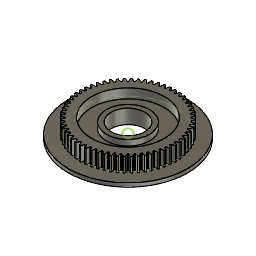
roller (Autodesk Fusion 360 design; units mm, degrees)
part number: 2025-11-25-15-03-10-225
description: Spur Gear; Module: 1.617; Num Teeth: 60; Pressure Angle: 20.0; Backlash: 0.00 mm
part number: 2025-11-25-15-09-40-850
Autodesk Fusion 360 part; units mm, degrees
(part 1 of 11)
sketch "Sketch1" plane through (0, 0, 0) normal (0, 0, 1) x (1, 0, 0) in component "Spur Gear (60 teeth)"
  circle A0 centre (0, 0) radius 46.5188
  circle A1 centre (0, 0) radius 17.65
  dimension "d15" = 35.3
  measures "d15" diameter of A1
extrude "Extrude1" add sketch "Sketch1" along normal blind 15 in component "Spur Gear (60 teeth)"
sketch "Sketch2" plane through (0, 0, 0) normal (0, 0, 1) x (1, 0, 0) in component "Spur Gear (60 teeth)"
  spline S0 degree 5 poles (45.546, -1.8723) (45.5592, -1.8723) (45.5856, -1.8721) (45.6253, -1.8716) (45.6781, -1.8704) (45.7442, -1.8678) (45.8102, -1.8642) (45.8763, -1.8596) (45.9424, -1.8541) (46.0085, -1.8477) (46.0745, -1.8406) (46.1406, -1.8328) (46.2066, -1.8243) (46.2727, -1.8154) (46.3387, -1.806) (46.4047, -1.796) (46.4707, -1.7856) (46.5367, -1.7747) (46.6026, -1.7633) (46.6686, -1.7514) (46.7345, -1.739) (46.8004, -1.7263) (46.8663, -1.7131) (46.9322, -1.6994) (46.998, -1.6854) (47.0638, -1.671) (47.1296, -1.6562) (47.1954, -1.6411) (47.2611, -1.6255) (47.3268, -1.6096) (47.3925, -1.5933) (47.4582, -1.5767) (47.5239, -1.5597) (47.5895, -1.5424) (47.6551, -1.5247) (47.7206, -1.5067) (47.7862, -1.4884) (47.8517, -1.4697) (47.9171, -1.4507) (47.9826, -1.4314) (48.048, -1.4118) (48.1134, -1.3919) (48.1787, -1.3717) (48.2441, -1.3511) (48.3093, -1.3303) (48.3746, -1.3092) (48.4398, -1.2877) (48.505, -1.266) (48.5702, -1.244) (48.6353, -1.2217) (48.7004, -1.1991) (48.7654, -1.1763) (48.8305, -1.1532) (48.8955, -1.1297) (48.9604, -1.1061) (49.0253, -1.0821) (49.0902, -1.0579) (49.155, -1.0334) (49.2198, -1.0086) (49.2846, -0.9836) (49.3493, -0.9583) (49.414, -0.9328) (49.4787, -0.907) (49.5433, -0.881) (49.6079, -0.8546) (49.6724, -0.8281) (49.7369, -0.8013) (49.8013, -0.7742) (49.8657, -0.7469) (49.9301, -0.7194) (49.9944, -0.6916) (50.0459, -0.6691) (50.0844, -0.6522) (50.1101, -0.6409) (50.123, -0.6352) knots 0 0 0 0 0 0 0.01428571 0.02857143 0.04285714 0.05714286 0.07142857 0.08571429 0.1 0.11428571 0.12857143 0.14285714 0.15714286 0.17142857 0.18571429 0.2 0.21428571 0.22857143 0.24285714 0.25714286 0.27142857 0.28571429 0.3 0.31428571 0.32857143 0.34285714 0.35714286 0.37142857 0.38571429 0.4 0.41428571 0.42857143 0.44285714 0.45714286 0.47142857 0.48571429 0.5 0.51428571 0.52857143 0.54285714 0.55714286 0.57142857 0.58571429 0.6 0.61428571 0.62857143 0.64285714 0.65714286 0.67142857 0.68571429 0.7 0.71428571 0.72857143 0.74285714 0.75714286 0.77142857 0.78571429 0.8 0.81428571 0.82857143 0.84285714 0.85714286 0.87142857 0.88571429 0.9 0.91428571 0.92857143 0.94285714 0.95714286 0.97142857 0.98571429 1 1 1 1 1 1
  spline S1 degree 5 poles (45.546, 1.8723) (45.5592, 1.8723) (45.5856, 1.8721) (45.6253, 1.8716) (45.6781, 1.8704) (45.7442, 1.8678) (45.8102, 1.8642) (45.8763, 1.8596) (45.9424, 1.8541) (46.0085, 1.8477) (46.0745, 1.8406) (46.1406, 1.8328) (46.2066, 1.8243) (46.2727, 1.8154) (46.3387, 1.806) (46.4047, 1.796) (46.4707, 1.7856) (46.5367, 1.7747) (46.6026, 1.7633) (46.6686, 1.7514) (46.7345, 1.739) (46.8004, 1.7263) (46.8663, 1.7131) (46.9322, 1.6994) (46.998, 1.6854) (47.0638, 1.671) (47.1296, 1.6562) (47.1954, 1.6411) (47.2611, 1.6255) (47.3268, 1.6096) (47.3925, 1.5933) (47.4582, 1.5767) (47.5239, 1.5597) (47.5895, 1.5424) (47.6551, 1.5247) (47.7206, 1.5067) (47.7862, 1.4884) (47.8517, 1.4697) (47.9171, 1.4507) (47.9826, 1.4314) (48.048, 1.4118) (48.1134, 1.3919) (48.1787, 1.3717) (48.2441, 1.3511) (48.3093, 1.3303) (48.3746, 1.3092) (48.4398, 1.2877) (48.505, 1.266) (48.5702, 1.244) (48.6353, 1.2217) (48.7004, 1.1991) (48.7654, 1.1763) (48.8305, 1.1532) (48.8955, 1.1297) (48.9604, 1.1061) (49.0253, 1.0821) (49.0902, 1.0579) (49.155, 1.0334) (49.2198, 1.0086) (49.2846, 0.9836) (49.3493, 0.9583) (49.414, 0.9328) (49.4787, 0.907) (49.5433, 0.881) (49.6079, 0.8546) (49.6724, 0.8281) (49.7369, 0.8013) (49.8013, 0.7742) (49.8657, 0.7469) (49.9301, 0.7194) (49.9944, 0.6916) (50.0459, 0.6691) (50.0844, 0.6522) (50.1101, 0.6409) (50.123, 0.6352) knots 0 0 0 0 0 0 0.01428571 0.02857143 0.04285714 0.05714286 0.07142857 0.08571429 0.1 0.11428571 0.12857143 0.14285714 0.15714286 0.17142857 0.18571429 0.2 0.21428571 0.22857143 0.24285714 0.25714286 0.27142857 0.28571429 0.3 0.31428571 0.32857143 0.34285714 0.35714286 0.37142857 0.38571429 0.4 0.41428571 0.42857143 0.44285714 0.45714286 0.47142857 0.48571429 0.5 0.51428571 0.52857143 0.54285714 0.55714286 0.57142857 0.58571429 0.6 0.61428571 0.62857143 0.64285714 0.65714286 0.67142857 0.68571429 0.7 0.71428571 0.72857143 0.74285714 0.75714286 0.77142857 0.78571429 0.8 0.81428571 0.82857143 0.84285714 0.85714286 0.87142857 0.88571429 0.9 0.91428571 0.92857143 0.94285714 0.95714286 0.97142857 0.98571429 1 1 1 1 1 1
  arc A0 (50.123, -0.6352) -> (50.123, 0.6352) centre (0, 0) ccw
  line L0 (45.546, 1.8723) -> (45.546, -1.8723)
  point P0 (45.8713, -1.8597)
  point P1 (46.1974, -1.8254)
  point P2 (46.524, -1.7767)
  point P3 (46.8509, -1.7161)
  point P4 (47.1781, -1.645)
  point P5 (47.5055, -1.5644)
  point P6 (47.833, -1.475)
  point P7 (48.1605, -1.3772)
  point P8 (48.488, -1.2716)
  point P9 (48.8154, -1.1585)
  point P10 (49.1426, -1.038)
  point P11 (49.4697, -0.9105)
  point P12 (49.7965, -0.7762)
  point P13 (45.8713, 1.8597)
  point P14 (46.1974, 1.8254)
  point P15 (46.524, 1.7767)
  point P16 (46.8509, 1.7161)
  point P17 (47.1781, 1.645)
  point P18 (47.5055, 1.5644)
  point P19 (47.833, 1.475)
  point P20 (48.1605, 1.3772)
  point P21 (48.488, 1.2716)
  point P22 (48.8154, 1.1585)
  point P23 (49.1426, 1.038)
  point P24 (49.4697, 0.9105)
  point P25 (49.7965, 0.7762)
extrude "Extrude2" add sketch "Sketch2" along normal blind 15 in component "Spur Gear (60 teeth)"
fillet "Fillet1" radius 0.4 2 edges at (46.4846, 1.7832, 7.5) (46.4846, -1.7832, 7.5) in component "Spur Gear (60 teeth)"
pattern_circular "C-Pattern1" count 60 over 360 about axis through (0, 0, 0) along (0, 0, 1) of "Extrude2", "Fillet1" in component "Spur Gear (60 teeth)"
sketch "Sketch3" plane through (0, 0, 0) normal (0, 0, 1) x (1, 0, 0) in component "Spur Gear (60 teeth)"
  circle A0 centre (0, 0) radius 48.51 construction
sketch "Sketch1 (2)" plane through (0, 0, 0) normal (0, 0, -1) x (1, 0, 0)
  circle A0 centre (0, 0) radius 17.65
  spline S0 degree 3 poles (46.1303, 8.0392) (46.0824, 8.0188) (46.039, 7.9892) (45.9659, 7.915) (45.9369, 7.8711) (45.9032, 7.7887) (45.894, 7.7528) (45.8858, 7.6794) (45.8868, 7.6424) (45.8928, 7.606) knots 0 0 0 0 0.015626 0.015626 0.031252 0.031252 0.042323 0.042323 0.053393 0.053393 0.053393 0.053393
  spline S1 degree 5 poles (46.1303, 8.0392) (46.1316, 8.0398) (46.1452, 8.0456) (46.1711, 8.0567) (46.2094, 8.0733) (46.2599, 8.0954) (46.3214, 8.1228) (46.3828, 8.1506) (46.4441, 8.1788) (46.5052, 8.2073) (46.5663, 8.2361) (46.6273, 8.2654) (46.6882, 8.295) (46.7489, 8.3249) (46.8096, 8.3552) (46.8702, 8.3857) (46.9307, 8.4167) (46.9911, 8.4479) (47.0514, 8.4795) (47.1116, 8.5113) (47.1717, 8.5435) (47.2317, 8.576) (47.2916, 8.6088) (47.3514, 8.6419) (47.4111, 8.6752) (47.4707, 8.7089) (47.5303, 8.7429) (47.5897, 8.7771) (47.649, 8.8116) (47.7083, 8.8464) (47.7674, 8.8815) (47.8265, 8.9168) (47.8855, 8.9524) (47.9444, 8.9883) (48.0032, 9.0245) (48.0619, 9.0609) (48.1205, 9.0975) (48.179, 9.1345) (48.2374, 9.1717) (48.2957, 9.2091) (48.354, 9.2468) (48.4121, 9.2847) (48.4702, 9.3229) (48.5281, 9.3613) (48.586, 9.4) (48.6438, 9.4389) (48.7015, 9.4781) (48.7591, 9.5175) (48.8166, 9.5571) (48.874, 9.597) (48.9314, 9.6371) (48.9886, 9.6774) (49.0457, 9.718) (49.0914, 9.7506) (49.1256, 9.7752) (49.1483, 9.7916) (49.1597, 9.7998) knots 0.269981 0.269981 0.269981 0.269981 0.269981 0.269981 0.271429 0.285714 0.3 0.314286 0.328571 0.342857 0.357143 0.371429 0.385714 0.4 0.414286 0.428571 0.442857 0.457143 0.471429 0.485714 0.5 0.514286 0.528571 0.542857 0.557143 0.571429 0.585714 0.6 0.614286 0.628571 0.642857 0.657143 0.671429 0.685714 0.7 0.714286 0.728571 0.742857 0.757143 0.771429 0.785714 0.8 0.814286 0.828571 0.842857 0.857143 0.871429 0.885714 0.9 0.914286 0.928571 0.942857 0.957143 0.971429 0.985714 1 1 1 1 1 1
  arc A1 (49.1597, 9.7998) -> (48.8956, 11.0425) centre (0, 0) ccw
  spline S2 degree 5 poles (45.412, 11.4187) (45.4134, 11.4187) (45.4282, 11.4189) (45.4564, 11.4193) (45.4981, 11.4197) (45.5532, 11.42) (45.6206, 11.42) (45.6879, 11.4196) (45.7554, 11.4188) (45.8229, 11.4177) (45.8904, 11.4161) (45.958, 11.4142) (46.0256, 11.412) (46.0933, 11.4093) (46.1611, 11.4064) (46.2289, 11.4031) (46.2967, 11.3994) (46.3646, 11.3954) (46.4325, 11.3911) (46.5004, 11.3865) (46.5684, 11.3816) (46.6364, 11.3763) (46.7045, 11.3707) (46.7726, 11.3648) (46.8407, 11.3586) (46.9089, 11.3521) (46.9771, 11.3453) (47.0453, 11.3382) (47.1136, 11.3308) (47.1818, 11.3231) (47.2502, 11.3151) (47.3185, 11.3069) (47.3869, 11.2983) (47.4552, 11.2895) (47.5237, 11.2804) (47.5921, 11.271) (47.6605, 11.2613) (47.729, 11.2514) (47.7975, 11.2412) (47.866, 11.2307) (47.9346, 11.22) (48.0031, 11.209) (48.0717, 11.1977) (48.1403, 11.1862) (48.2089, 11.1744) (48.2775, 11.1623) (48.3461, 11.15) (48.4148, 11.1375) (48.4834, 11.1246) (48.5521, 11.1116) (48.6208, 11.0983) (48.6895, 11.0847) (48.7582, 11.0709) (48.8131, 11.0596) (48.8544, 11.0511) (48.8819, 11.0453) (48.8956, 11.0425) knots 0.269981 0.269981 0.269981 0.269981 0.269981 0.269981 0.271429 0.285714 0.3 0.314286 0.328571 0.342857 0.357143 0.371429 0.385714 0.4 0.414286 0.428571 0.442857 0.457143 0.471429 0.485714 0.5 0.514286 0.528571 0.542857 0.557143 0.571429 0.585714 0.6 0.614286 0.628571 0.642857 0.657143 0.671429 0.685714 0.7 0.714286 0.728571 0.742857 0.757143 0.771429 0.785714 0.8 0.814286 0.828571 0.842857 0.857143 0.871429 0.885714 0.9 0.914286 0.928571 0.942857 0.957143 0.971429 0.985714 1 1 1 1 1 1
  spline S3 degree 3 poles (45.0188, 11.7179) (45.0319, 11.6675) (45.0547, 11.6201) (45.1173, 11.5368) (45.1564, 11.5017) (45.2328, 11.4561) (45.267, 11.4417) (45.3383, 11.4227) (45.3751, 11.4181) (45.412, 11.4187) knots 0 0 0 0 0.015626 0.015626 0.031252 0.031252 0.042323 0.042323 0.053393 0.053393 0.053393 0.053393
  arc A2 (45.0188, 11.7179) -> (44.8463, 12.3614) centre (0, 0) ccw
  spline S4 degree 3 poles (45.0373, 12.8171) (44.9918, 12.7918) (44.9517, 12.7578) (44.8867, 12.6763) (44.8625, 12.6297) (44.8376, 12.5442) (44.8322, 12.5076) (44.8317, 12.4337) (44.8365, 12.397) (44.8463, 12.3614) knots 0 0 0 0 0.015626 0.015626 0.031252 0.031252 0.042323 0.042323 0.053393 0.053393 0.053393 0.053393
  spline S5 degree 5 poles (45.0373, 12.8171) (45.0385, 12.8178) (45.0514, 12.825) (45.076, 12.8388) (45.1124, 12.8593) (45.1603, 12.8866) (45.2186, 12.9202) (45.2767, 12.9543) (45.3347, 12.9887) (45.3926, 13.0234) (45.4503, 13.0585) (45.5079, 13.094) (45.5654, 13.1298) (45.6227, 13.1659) (45.6798, 13.2023) (45.7369, 13.2391) (45.7938, 13.2762) (45.8506, 13.3135) (45.9073, 13.3512) (45.9638, 13.3892) (46.0202, 13.4275) (46.0765, 13.4661) (46.1326, 13.5049) (46.1887, 13.5441) (46.2446, 13.5835) (46.3003, 13.6232) (46.356, 13.6632) (46.4115, 13.7035) (46.4669, 13.744) (46.5222, 13.7848) (46.5774, 13.8259) (46.6325, 13.8672) (46.6874, 13.9088) (46.7422, 13.9506) (46.7969, 13.9927) (46.8515, 14.0351) (46.9059, 14.0777) (46.9602, 14.1205) (47.0145, 14.1636) (47.0686, 14.2069) (47.1225, 14.2505) (47.1764, 14.2943) (47.2301, 14.3383) (47.2838, 14.3826) (47.3373, 14.4271) (47.3907, 14.4719) (47.444, 14.5169) (47.4971, 14.5621) (47.5502, 14.6075) (47.6031, 14.6531) (47.656, 14.699) (47.7087, 14.7451) (47.7613, 14.7914) (47.8032, 14.8286) (47.8347, 14.8567) (47.8556, 14.8754) (47.8661, 14.8847) knots 0.269981 0.269981 0.269981 0.269981 0.269981 0.269981 0.271429 0.285714 0.3 0.314286 0.328571 0.342857 0.357143 0.371429 0.385714 0.4 0.414286 0.428571 0.442857 0.457143 0.471429 0.485714 0.5 0.514286 0.528571 0.542857 0.557143 0.571429 0.585714 0.6 0.614286 0.628571 0.642857 0.657143 0.671429 0.685714 0.7 0.714286 0.728571 0.742857 0.757143 0.771429 0.785714 0.8 0.814286 0.828571 0.842857 0.857143 0.871429 0.885714 0.9 0.914286 0.928571 0.942857 0.957143 0.971429 0.985714 1 1 1 1 1 1
  arc A3 (47.8661, 14.8847) -> (47.4735, 16.093) centre (0, 0) ccw
  spline S6 degree 5 poles (43.9697, 16.103) (43.971, 16.1031) (43.9857, 16.1049) (44.0137, 16.1082) (44.0551, 16.113) (44.11, 16.1191) (44.1769, 16.1261) (44.244, 16.1328) (44.3111, 16.139) (44.3784, 16.1449) (44.4457, 16.1504) (44.5131, 16.1556) (44.5806, 16.1604) (44.6482, 16.1649) (44.7159, 16.169) (44.7837, 16.1728) (44.8515, 16.1763) (44.9194, 16.1794) (44.9874, 16.1823) (45.0555, 16.1847) (45.1236, 16.1869) (45.1918, 16.1888) (45.2601, 16.1904) (45.3284, 16.1916) (45.3968, 16.1926) (45.4653, 16.1932) (45.5338, 16.1936) (45.6024, 16.1937) (45.6711, 16.1934) (45.7398, 16.1929) (45.8086, 16.1921) (45.8774, 16.1911) (45.9463, 16.1897) (46.0152, 16.1881) (46.0842, 16.1862) (46.1532, 16.184) (46.2223, 16.1815) (46.2915, 16.1788) (46.3606, 16.1758) (46.4299, 16.1726) (46.4992, 16.169) (46.5685, 16.1653) (46.6379, 16.1612) (46.7073, 16.1569) (46.7767, 16.1524) (46.8462, 16.1476) (46.9158, 16.1425) (46.9854, 16.1372) (47.055, 16.1316) (47.1246, 16.1258) (47.1943, 16.1197) (47.2641, 16.1134) (47.3338, 16.1069) (47.3897, 16.1014) (47.4316, 16.0972) (47.4595, 16.0944) (47.4735, 16.093) knots 0.269981 0.269981 0.269981 0.269981 0.269981 0.269981 0.271429 0.285714 0.3 0.314286 0.328571 0.342857 0.357143 0.371429 0.385714 0.4 0.414286 0.428571 0.442857 0.457143 0.471429 0.485714 0.5 0.514286 0.528571 0.542857 0.557143 0.571429 0.585714 0.6 0.614286 0.628571 0.642857 0.657143 0.671429 0.685714 0.7 0.714286 0.728571 0.742857 0.757143 0.771429 0.785714 0.8 0.814286 0.828571 0.842857 0.857143 0.871429 0.885714 0.9 0.914286 0.928571 0.942857 0.957143 0.971429 0.985714 1 1 1 1 1 1
  spline S7 degree 3 poles (43.5473, 16.3594) (43.5656, 16.3107) (43.5933, 16.266) (43.6642, 16.1896) (43.7068, 16.1588) (43.7876, 16.1215) (43.823, 16.1107) (43.896, 16.0992) (43.933, 16.0986) (43.9697, 16.103) knots 0 0 0 0 0.015626 0.015626 0.031252 0.031252 0.042323 0.042323 0.053393 0.053393 0.053393 0.053393
  arc A4 (43.5473, 16.3594) -> (43.3086, 16.9814) centre (0, 0) ccw
  spline S8 degree 3 poles (43.4508, 17.4546) (43.4082, 17.4246) (43.3719, 17.3866) (43.3158, 17.2988) (43.2966, 17.2499) (43.2808, 17.1623) (43.2793, 17.1253) (43.2864, 17.0518) (43.2951, 17.0158) (43.3086, 16.9814) knots 0 0 0 0 0.015626 0.015626 0.031252 0.031252 0.042323 0.042323 0.053393 0.053393 0.053393 0.053393
  spline S9 degree 5 poles (43.4508, 17.4546) (43.4519, 17.4554) (43.464, 17.4639) (43.4871, 17.4802) (43.5211, 17.5043) (43.5659, 17.5365) (43.6203, 17.5761) (43.6746, 17.616) (43.7287, 17.6563) (43.7826, 17.6969) (43.8363, 17.7378) (43.8899, 17.7791) (43.9433, 17.8207) (43.9965, 17.8626) (44.0496, 17.9048) (44.1025, 17.9474) (44.1552, 17.9902) (44.2078, 18.0333) (44.2602, 18.0767) (44.3125, 18.1204) (44.3645, 18.1644) (44.4165, 18.2086) (44.4683, 18.2531) (44.5199, 18.2979) (44.5714, 18.343) (44.6227, 18.3883) (44.6739, 18.4339) (44.7249, 18.4797) (44.7758, 18.5258) (44.8265, 18.5722) (44.8771, 18.6188) (44.9275, 18.6657) (44.9778, 18.7128) (45.0279, 18.7601) (45.0779, 18.8077) (45.1277, 18.8555) (45.1774, 18.9036) (45.227, 18.9518) (45.2764, 19.0004) (45.3257, 19.0491) (45.3748, 19.0981) (45.4238, 19.1473) (45.4727, 19.1967) (45.5214, 19.2463) (45.5699, 19.2962) (45.6184, 19.3463) (45.6666, 19.3966) (45.7148, 19.4471) (45.7628, 19.4978) (45.8107, 19.5487) (45.8584, 19.5999) (45.906, 19.6512) (45.9535, 19.7028) (45.9914, 19.7442) (46.0197, 19.7754) (46.0385, 19.7962) (46.048, 19.8066) knots 0.269981 0.269981 0.269981 0.269981 0.269981 0.269981 0.271429 0.285714 0.3 0.314286 0.328571 0.342857 0.357143 0.371429 0.385714 0.4 0.414286 0.428571 0.442857 0.457143 0.471429 0.485714 0.5 0.514286 0.528571 0.542857 0.557143 0.571429 0.585714 0.6 0.614286 0.628571 0.642857 0.657143 0.671429 0.685714 0.7 0.714286 0.728571 0.742857 0.757143 0.771429 0.785714 0.8 0.814286 0.828571 0.842857 0.857143 0.871429 0.885714 0.9 0.914286 0.928571 0.942857 0.957143 0.971429 0.985714 1 1 1 1 1 1
  arc A5 (46.048, 19.8066) -> (45.5313, 20.9671) centre (0, 0) ccw
  spline S10 degree 5 poles (42.0456, 20.6108) (42.0469, 20.6112) (42.0613, 20.6144) (42.0889, 20.6207) (42.1295, 20.6298) (42.1834, 20.6415) (42.2493, 20.6555) (42.3153, 20.6691) (42.3814, 20.6824) (42.4476, 20.6953) (42.514, 20.7078) (42.5805, 20.72) (42.6472, 20.7319) (42.7139, 20.7434) (42.7808, 20.7545) (42.8478, 20.7654) (42.9149, 20.7759) (42.9821, 20.7862) (43.0495, 20.7961) (43.1169, 20.8057) (43.1844, 20.815) (43.2521, 20.8239) (43.3198, 20.8326) (43.3876, 20.841) (43.4556, 20.8491) (43.5236, 20.8569) (43.5917, 20.8645) (43.6599, 20.8717) (43.7282, 20.8787) (43.7966, 20.8853) (43.8651, 20.8917) (43.9336, 20.8979) (44.0023, 20.9037) (44.071, 20.9093) (44.1398, 20.9146) (44.2087, 20.9197) (44.2777, 20.9244) (44.3467, 20.929) (44.4158, 20.9332) (44.485, 20.9372) (44.5543, 20.941) (44.6237, 20.9444) (44.6931, 20.9477) (44.7626, 20.9507) (44.8321, 20.9534) (44.9017, 20.9559) (44.9714, 20.9581) (45.0412, 20.9601) (45.111, 20.9618) (45.1809, 20.9633) (45.2508, 20.9646) (45.3208, 20.9656) (45.3909, 20.9664) (45.447, 20.9668) (45.4891, 20.967) (45.5172, 20.9671) (45.5313, 20.9671) knots 0.269981 0.269981 0.269981 0.269981 0.269981 0.269981 0.271429 0.285714 0.3 0.314286 0.328571 0.342857 0.357143 0.371429 0.385714 0.4 0.414286 0.428571 0.442857 0.457143 0.471429 0.485714 0.5 0.514286 0.528571 0.542857 0.557143 0.571429 0.585714 0.6 0.614286 0.628571 0.642857 0.657143 0.671429 0.685714 0.7 0.714286 0.728571 0.742857 0.757143 0.771429 0.785714 0.8 0.814286 0.828571 0.842857 0.857143 0.871429 0.885714 0.9 0.914286 0.928571 0.942857 0.957143 0.971429 0.985714 1 1 1 1 1 1
  spline S11 degree 3 poles (41.5987, 20.8217) (41.622, 20.7752) (41.6542, 20.7336) (41.7327, 20.6651) (41.7783, 20.6389) (41.8625, 20.6102) (41.899, 20.6032) (41.9727, 20.5994) (42.0096, 20.6026) (42.0456, 20.6108) knots 0 0 0 0 0.015626 0.015626 0.031252 0.031252 0.042323 0.042323 0.053393 0.053393 0.053393 0.053393
  arc A6 (41.5987, 20.8217) -> (41.2963, 21.4154) centre (0, 0) ccw
  spline S12 degree 3 poles (41.3883, 21.9008) (41.3491, 21.8666) (41.3169, 21.825) (41.2703, 21.7318) (41.2563, 21.6811) (41.2497, 21.5924) (41.2521, 21.5554) (41.2669, 21.4831) (41.2793, 21.4481) (41.2963, 21.4154) knots 0 0 0 0 0.015626 0.015626 0.031252 0.031252 0.042323 0.042323 0.053393 0.053393 0.053393 0.053393
  spline S13 degree 5 poles (41.3883, 21.9008) (41.3893, 21.9017) (41.4005, 21.9115) (41.4217, 21.9301) (41.453, 21.9576) (41.4942, 21.9943) (41.5442, 22.0394) (41.594, 22.0848) (41.6436, 22.1305) (41.6929, 22.1765) (41.7421, 22.2228) (41.7911, 22.2695) (41.8398, 22.3164) (41.8884, 22.3637) (41.9367, 22.4112) (41.9849, 22.459) (42.0328, 22.5071) (42.0806, 22.5555) (42.1282, 22.6041) (42.1756, 22.653) (42.2228, 22.7022) (42.2698, 22.7516) (42.3167, 22.8013) (42.3634, 22.8513) (42.4098, 22.9015) (42.4561, 22.9519) (42.5023, 23.0026) (42.5482, 23.0535) (42.594, 23.1047) (42.6396, 23.1561) (42.685, 23.2077) (42.7303, 23.2596) (42.7754, 23.3117) (42.8203, 23.364) (42.865, 23.4166) (42.9096, 23.4693) (42.954, 23.5223) (42.9982, 23.5755) (43.0423, 23.6289) (43.0862, 23.6826) (43.13, 23.7364) (43.1735, 23.7905) (43.2169, 23.8447) (43.2602, 23.8992) (43.3033, 23.9538) (43.3462, 24.0087) (43.389, 24.0638) (43.4316, 24.1191) (43.474, 24.1745) (43.5163, 24.2302) (43.5585, 24.286) (43.6004, 24.3421) (43.6422, 24.3983) (43.6756, 24.4434) (43.7005, 24.4774) (43.7171, 24.5001) (43.7254, 24.5114) knots 0.269981 0.269981 0.269981 0.269981 0.269981 0.269981 0.271429 0.285714 0.3 0.314286 0.328571 0.342857 0.357143 0.371429 0.385714 0.4 0.414286 0.428571 0.442857 0.457143 0.471429 0.485714 0.5 0.514286 0.528571 0.542857 0.557143 0.571429 0.585714 0.6 0.614286 0.628571 0.642857 0.657143 0.671429 0.685714 0.7 0.714286 0.728571 0.742857 0.757143 0.771429 0.785714 0.8 0.814286 0.828571 0.842857 0.857143 0.871429 0.885714 0.9 0.914286 0.928571 0.942857 0.957143 0.971429 0.985714 1 1 1 1 1 1
  arc A7 (43.7254, 24.5114) -> (43.0902, 25.6116) centre (0, 0) ccw
  spline S14 degree 5 poles (39.6608, 24.8929) (39.6621, 24.8933) (39.6761, 24.8981) (39.7028, 24.9072) (39.7424, 24.9205) (39.7947, 24.9378) (39.8587, 24.9586) (39.923, 24.9791) (39.9873, 24.9991) (40.0519, 25.0189) (40.1166, 25.0383) (40.1815, 25.0574) (40.2465, 25.0761) (40.3117, 25.0946) (40.377, 25.1127) (40.4425, 25.1305) (40.5081, 25.148) (40.5739, 25.1651) (40.6398, 25.182) (40.7059, 25.1986) (40.7721, 25.2149) (40.8384, 25.2309) (40.9049, 25.2467) (40.9715, 25.2621) (41.0382, 25.2773) (41.105, 25.2921) (41.172, 25.3067) (41.2391, 25.3211) (41.3063, 25.3351) (41.3736, 25.3489) (41.441, 25.3624) (41.5085, 25.3757) (41.5762, 25.3887) (41.644, 25.4014) (41.7118, 25.4139) (41.7798, 25.4261) (41.8479, 25.4381) (41.9161, 25.4498) (41.9844, 25.4613) (42.0528, 25.4725) (42.1213, 25.4834) (42.1899, 25.4941) (42.2586, 25.5046) (42.3274, 25.5148) (42.3963, 25.5248) (42.4653, 25.5346) (42.5343, 25.5441) (42.6035, 25.5533) (42.6728, 25.5624) (42.7421, 25.5712) (42.8115, 25.5797) (42.8811, 25.588) (42.9507, 25.5961) (43.0064, 25.6024) (43.0483, 25.607) (43.0762, 25.6101) (43.0902, 25.6116) knots 0.269981 0.269981 0.269981 0.269981 0.269981 0.269981 0.271429 0.285714 0.3 0.314286 0.328571 0.342857 0.357143 0.371429 0.385714 0.4 0.414286 0.428571 0.442857 0.457143 0.471429 0.485714 0.5 0.514286 0.528571 0.542857 0.557143 0.571429 0.585714 0.6 0.614286 0.628571 0.642857 0.657143 0.671429 0.685714 0.7 0.714286 0.728571 0.742857 0.757143 0.771429 0.785714 0.8 0.814286 0.828571 0.842857 0.857143 0.871429 0.885714 0.9 0.914286 0.928571 0.942857 0.957143 0.971429 0.985714 1 1 1 1 1 1
  spline S15 degree 3 poles (39.1944, 25.0559) (39.2224, 25.012) (39.2588, 24.9741) (39.344, 24.9142) (39.3921, 24.8928) (39.4789, 24.8731) (39.5158, 24.87) (39.5895, 24.8739) (39.6259, 24.881) (39.6608, 24.8929) knots 0 0 0 0 0.015626 0.015626 0.031252 0.031252 0.042323 0.042323 0.053393 0.053393 0.053393 0.053393
  arc A8 (39.1944, 25.0559) -> (38.8315, 25.6147) centre (0, 0) ccw
  spline S16 degree 3 poles (38.8723, 26.1071) (38.8369, 26.0689) (38.8092, 26.0242) (38.7726, 25.9267) (38.764, 25.8748) (38.7667, 25.7859) (38.773, 25.7493) (38.7952, 25.679) (38.8112, 25.6455) (38.8315, 25.6147) knots 0 0 0 0 0.015626 0.015626 0.031252 0.031252 0.042323 0.042323 0.053393 0.053393 0.053393 0.053393
  spline S17 degree 5 poles (38.8723, 26.1071) (38.8732, 26.1081) (38.8833, 26.119) (38.9025, 26.1397) (38.9307, 26.1704) (38.9678, 26.2112) (39.0128, 26.2612) (39.0576, 26.3115) (39.1022, 26.3622) (39.1465, 26.4131) (39.1905, 26.4643) (39.2343, 26.5158) (39.2779, 26.5676) (39.3213, 26.6197) (39.3644, 26.672) (39.4073, 26.7246) (39.4499, 26.7774) (39.4924, 26.8305) (39.5347, 26.8839) (39.5767, 26.9375) (39.6185, 26.9913) (39.6601, 27.0454) (39.7015, 27.0997) (39.7427, 27.1543) (39.7837, 27.2091) (39.8244, 27.2641) (39.865, 27.3193) (39.9054, 27.3747) (39.9456, 27.4304) (39.9855, 27.4863) (40.0253, 27.5424) (40.0649, 27.5987) (40.1043, 27.6552) (40.1435, 27.712) (40.1825, 27.7689) (40.2213, 27.826) (40.2599, 27.8834) (40.2984, 27.9409) (40.3366, 27.9986) (40.3747, 28.0566) (40.4126, 28.1147) (40.4502, 28.173) (40.4877, 28.2315) (40.5251, 28.2902) (40.5622, 28.3491) (40.5992, 28.4081) (40.6359, 28.4673) (40.6725, 28.5268) (40.709, 28.5864) (40.7452, 28.6461) (40.7813, 28.7061) (40.8171, 28.7662) (40.8529, 28.8265) (40.8813, 28.8749) (40.9025, 28.9112) (40.9166, 28.9355) (40.9237, 28.9477) knots 0.269981 0.269981 0.269981 0.269981 0.269981 0.269981 0.271429 0.285714 0.3 0.314286 0.328571 0.342857 0.357143 0.371429 0.385714 0.4 0.414286 0.428571 0.442857 0.457143 0.471429 0.485714 0.5 0.514286 0.528571 0.542857 0.557143 0.571429 0.585714 0.6 0.614286 0.628571 0.642857 0.657143 0.671429 0.685714 0.7 0.714286 0.728571 0.742857 0.757143 0.771429 0.785714 0.8 0.814286 0.828571 0.842857 0.857143 0.871429 0.885714 0.9 0.914286 0.928571 0.942857 0.957143 0.971429 0.985714 1 1 1 1 1 1
  arc A9 (40.9237, 28.9477) -> (40.177, 29.9754) centre (0, 0) ccw
  spline S18 degree 5 poles (36.8415, 28.9022) (36.8428, 28.9028) (36.8562, 28.909) (36.8818, 28.9208) (36.9197, 28.9382) (36.97, 28.9609) (37.0315, 28.9883) (37.0932, 29.0153) (37.1551, 29.042) (37.2173, 29.0684) (37.2796, 29.0945) (37.3421, 29.1202) (37.4048, 29.1457) (37.4678, 29.1708) (37.5308, 29.1956) (37.5941, 29.2202) (37.6576, 29.2444) (37.7212, 29.2684) (37.785, 29.2921) (37.8489, 29.3155) (37.9131, 29.3386) (37.9774, 29.3615) (38.0418, 29.3841) (38.1064, 29.4064) (38.1712, 29.4284) (38.2361, 29.4502) (38.3012, 29.4717) (38.3664, 29.493) (38.4317, 29.514) (38.4972, 29.5348) (38.5629, 29.5553) (38.6287, 29.5755) (38.6946, 29.5955) (38.7607, 29.6153) (38.8269, 29.6348) (38.8932, 29.654) (38.9597, 29.673) (39.0263, 29.6918) (39.093, 29.7103) (39.1598, 29.7286) (39.2268, 29.7467) (39.2939, 29.7645) (39.3611, 29.7821) (39.4285, 29.7995) (39.496, 29.8166) (39.5635, 29.8335) (39.6313, 29.8502) (39.6991, 29.8666) (39.767, 29.8829) (39.8351, 29.8988) (39.9032, 29.9146) (39.9715, 29.9302) (40.0399, 29.9455) (40.0947, 29.9576) (40.1358, 29.9665) (40.1633, 29.9725) (40.177, 29.9754) knots 0.269981 0.269981 0.269981 0.269981 0.269981 0.269981 0.271429 0.285714 0.3 0.314286 0.328571 0.342857 0.357143 0.371429 0.385714 0.4 0.414286 0.428571 0.442857 0.457143 0.471429 0.485714 0.5 0.514286 0.528571 0.542857 0.557143 0.571429 0.585714 0.6 0.614286 0.628571 0.642857 0.657143 0.671429 0.685714 0.7 0.714286 0.728571 0.742857 0.757143 0.771429 0.785714 0.8 0.814286 0.828571 0.842857 0.857143 0.871429 0.885714 0.9 0.914286 0.928571 0.942857 0.957143 0.971429 0.985714 1 1 1 1 1 1
  spline S19 degree 3 poles (36.3606, 29.0156) (36.3931, 28.9749) (36.4332, 28.9409) (36.5242, 28.8903) (36.5743, 28.8741) (36.6626, 28.8635) (36.6997, 28.8643) (36.7726, 28.8759) (36.8081, 28.8867) (36.8415, 28.9022) knots 0 0 0 0 0.015626 0.015626 0.031252 0.031252 0.042323 0.042323 0.053393 0.053393 0.053393 0.053393
  arc A10 (36.3606, 29.0156) -> (35.9413, 29.5334) centre (0, 0) ccw
  spline S20 degree 3 poles (35.9304, 30.0274) (35.8992, 29.9857) (35.8763, 29.9383) (35.8501, 29.8375) (35.847, 29.785) (35.859, 29.6968) (35.869, 29.6611) (35.8985, 29.5935) (35.9179, 29.5619) (35.9413, 29.5334) knots 0 0 0 0 0.015626 0.015626 0.031252 0.031252 0.042323 0.042323 0.053393 0.053393 0.053393 0.053393
  spline S21 degree 5 poles (35.9304, 30.0274) (35.9312, 30.0284) (35.9401, 30.0403) (35.957, 30.0629) (35.9819, 30.0964) (36.0145, 30.1408) (36.0541, 30.1953) (36.0934, 30.25) (36.1324, 30.305) (36.1711, 30.3603) (36.2095, 30.4159) (36.2477, 30.4717) (36.2857, 30.5277) (36.3233, 30.584) (36.3607, 30.6406) (36.3979, 30.6974) (36.4348, 30.7544) (36.4715, 30.8116) (36.5079, 30.8691) (36.5441, 30.9268) (36.5801, 30.9847) (36.6158, 31.0429) (36.6513, 31.1012) (36.6866, 31.1598) (36.7216, 31.2185) (36.7564, 31.2775) (36.791, 31.3367) (36.8253, 31.396) (36.8595, 31.4556) (36.8934, 31.5154) (36.9271, 31.5753) (36.9606, 31.6355) (36.9938, 31.6958) (37.0269, 31.7563) (37.0597, 31.817) (37.0924, 31.8779) (37.1248, 31.9389) (37.157, 32.0002) (37.189, 32.0616) (37.2208, 32.1232) (37.2524, 32.1849) (37.2838, 32.2469) (37.315, 32.309) (37.3459, 32.3712) (37.3767, 32.4337) (37.4073, 32.4963) (37.4377, 32.559) (37.4679, 32.6219) (37.4979, 32.685) (37.5277, 32.7482) (37.5573, 32.8116) (37.5867, 32.8752) (37.6159, 32.9389) (37.6391, 32.99) (37.6564, 33.0283) (37.6679, 33.054) (37.6737, 33.0668) knots 0.269981 0.269981 0.269981 0.269981 0.269981 0.269981 0.271429 0.285714 0.3 0.314286 0.328571 0.342857 0.357143 0.371429 0.385714 0.4 0.414286 0.428571 0.442857 0.457143 0.471429 0.485714 0.5 0.514286 0.528571 0.542857 0.557143 0.571429 0.585714 0.6 0.614286 0.628571 0.642857 0.657143 0.671429 0.685714 0.7 0.714286 0.728571 0.742857 0.757143 0.771429 0.785714 0.8 0.814286 0.828571 0.842857 0.857143 0.871429 0.885714 0.9 0.914286 0.928571 0.942857 0.957143 0.971429 0.985714 1 1 1 1 1 1
  arc A11 (37.6737, 33.0668) -> (36.8236, 34.0109) centre (0, 0) ccw
  spline S22 degree 5 poles (33.6186, 32.5949) (33.6198, 32.5956) (33.6325, 32.6032) (33.6567, 32.6176) (33.6926, 32.6388) (33.7402, 32.6667) (33.7986, 32.7003) (33.8571, 32.7336) (33.9159, 32.7667) (33.9749, 32.7994) (34.0342, 32.8319) (34.0937, 32.864) (34.1534, 32.8959) (34.2133, 32.9274) (34.2735, 32.9587) (34.3338, 32.9898) (34.3944, 33.0205) (34.4552, 33.051) (34.5161, 33.0812) (34.5773, 33.1112) (34.6386, 33.1409) (34.7002, 33.1704) (34.7619, 33.1996) (34.8239, 33.2285) (34.886, 33.2572) (34.9482, 33.2857) (35.0107, 33.3139) (35.0733, 33.3418) (35.1361, 33.3695) (35.1991, 33.397) (35.2623, 33.4243) (35.3256, 33.4513) (35.3891, 33.4781) (35.4527, 33.5046) (35.5165, 33.5309) (35.5805, 33.557) (35.6446, 33.5829) (35.7088, 33.6085) (35.7733, 33.6339) (35.8378, 33.6591) (35.9026, 33.6841) (35.9674, 33.7088) (36.0324, 33.7333) (36.0976, 33.7576) (36.1629, 33.7817) (36.2284, 33.8056) (36.294, 33.8293) (36.3597, 33.8527) (36.4255, 33.8759) (36.4916, 33.899) (36.5577, 33.9218) (36.624, 33.9444) (36.6904, 33.9668) (36.7436, 33.9845) (36.7836, 33.9977) (36.8103, 34.0065) (36.8236, 34.0109) knots 0.269981 0.269981 0.269981 0.269981 0.269981 0.269981 0.271429 0.285714 0.3 0.314286 0.328571 0.342857 0.357143 0.371429 0.385714 0.4 0.414286 0.428571 0.442857 0.457143 0.471429 0.485714 0.5 0.514286 0.528571 0.542857 0.557143 0.571429 0.585714 0.6 0.614286 0.628571 0.642857 0.657143 0.671429 0.685714 0.7 0.714286 0.728571 0.742857 0.757143 0.771429 0.785714 0.8 0.814286 0.828571 0.842857 0.857143 0.871429 0.885714 0.9 0.914286 0.928571 0.942857 0.957143 0.971429 0.985714 1 1 1 1 1 1
  spline S23 degree 3 poles (33.1285, 32.6574) (33.165, 32.6203) (33.2085, 32.5907) (33.3043, 32.5498) (33.3558, 32.5389) (33.4447, 32.5377) (33.4815, 32.5423) (33.5528, 32.5615) (33.5869, 32.5759) (33.6186, 32.5949) knots 0 0 0 0 0.015626 0.015626 0.031252 0.031252 0.042323 0.042323 0.053393 0.053393 0.053393 0.053393
  arc A12 (33.1285, 32.6574) -> (32.6574, 33.1285) centre (0, 0) ccw
  spline S24 degree 3 poles (32.5949, 33.6186) (32.5681, 33.5739) (32.5504, 33.5244) (32.5349, 33.4214) (32.5373, 33.3689) (32.5584, 33.2824) (32.5721, 33.248) (32.6085, 33.1838) (32.6311, 33.1544) (32.6574, 33.1285) knots 0 0 0 0 0.015626 0.015626 0.031252 0.031252 0.042323 0.042323 0.053393 0.053393 0.053393 0.053393
  spline S25 degree 5 poles (32.5949, 33.6186) (32.5956, 33.6198) (32.6032, 33.6325) (32.6176, 33.6567) (32.6388, 33.6926) (32.6667, 33.7402) (32.7003, 33.7986) (32.7336, 33.8571) (32.7667, 33.9159) (32.7994, 33.9749) (32.8319, 34.0342) (32.864, 34.0937) (32.8959, 34.1534) (32.9274, 34.2133) (32.9587, 34.2735) (32.9898, 34.3338) (33.0205, 34.3944) (33.051, 34.4552) (33.0812, 34.5161) (33.1112, 34.5773) (33.1409, 34.6386) (33.1704, 34.7002) (33.1996, 34.7619) (33.2285, 34.8239) (33.2572, 34.886) (33.2857, 34.9482) (33.3139, 35.0107) (33.3418, 35.0733) (33.3695, 35.1361) (33.397, 35.1991) (33.4243, 35.2623) (33.4513, 35.3256) (33.4781, 35.3891) (33.5046, 35.4527) (33.5309, 35.5165) (33.557, 35.5805) (33.5829, 35.6446) (33.6085, 35.7088) (33.6339, 35.7733) (33.6591, 35.8378) (33.6841, 35.9026) (33.7088, 35.9674) (33.7333, 36.0324) (33.7576, 36.0976) (33.7817, 36.1629) (33.8056, 36.2284) (33.8293, 36.294) (33.8527, 36.3597) (33.8759, 36.4255) (33.899, 36.4916) (33.9218, 36.5577) (33.9444, 36.624) (33.9668, 36.6904) (33.9845, 36.7436) (33.9977, 36.7836) (34.0065, 36.8103) (34.0109, 36.8236) knots 0.269981 0.269981 0.269981 0.269981 0.269981 0.269981 0.271429 0.285714 0.3 0.314286 0.328571 0.342857 0.357143 0.371429 0.385714 0.4 0.414286 0.428571 0.442857 0.457143 0.471429 0.485714 0.5 0.514286 0.528571 0.542857 0.557143 0.571429 0.585714 0.6 0.614286 0.628571 0.642857 0.657143 0.671429 0.685714 0.7 0.714286 0.728571 0.742857 0.757143 0.771429 0.785714 0.8 0.814286 0.828571 0.842857 0.857143 0.871429 0.885714 0.9 0.914286 0.928571 0.942857 0.957143 0.971429 0.985714 1 1 1 1 1 1
  arc A13 (34.0109, 36.8236) -> (33.0668, 37.6737) centre (0, 0) ccw
  spline S26 degree 5 poles (30.0274, 35.9304) (30.0284, 35.9312) (30.0403, 35.9401) (30.0629, 35.957) (30.0964, 35.9819) (30.1408, 36.0145) (30.1953, 36.0541) (30.25, 36.0934) (30.305, 36.1324) (30.3603, 36.1711) (30.4159, 36.2095) (30.4717, 36.2477) (30.5277, 36.2857) (30.584, 36.3233) (30.6406, 36.3607) (30.6974, 36.3979) (30.7544, 36.4348) (30.8116, 36.4715) (30.8691, 36.5079) (30.9268, 36.5441) (30.9847, 36.5801) (31.0429, 36.6158) (31.1012, 36.6513) (31.1598, 36.6866) (31.2185, 36.7216) (31.2775, 36.7564) (31.3367, 36.791) (31.396, 36.8253) (31.4556, 36.8595) (31.5154, 36.8934) (31.5753, 36.9271) (31.6355, 36.9606) (31.6958, 36.9938) (31.7563, 37.0269) (31.817, 37.0597) (31.8779, 37.0924) (31.9389, 37.1248) (32.0002, 37.157) (32.0616, 37.189) (32.1232, 37.2208) (32.1849, 37.2524) (32.2469, 37.2838) (32.309, 37.315) (32.3712, 37.3459) (32.4337, 37.3767) (32.4963, 37.4073) (32.559, 37.4377) (32.6219, 37.4679) (32.685, 37.4979) (32.7482, 37.5277) (32.8116, 37.5573) (32.8752, 37.5867) (32.9389, 37.6159) (32.99, 37.6391) (33.0283, 37.6564) (33.054, 37.6679) (33.0668, 37.6737) knots 0.269981 0.269981 0.269981 0.269981 0.269981 0.269981 0.271429 0.285714 0.3 0.314286 0.328571 0.342857 0.357143 0.371429 0.385714 0.4 0.414286 0.428571 0.442857 0.457143 0.471429 0.485714 0.5 0.514286 0.528571 0.542857 0.557143 0.571429 0.585714 0.6 0.614286 0.628571 0.642857 0.657143 0.671429 0.685714 0.7 0.714286 0.728571 0.742857 0.757143 0.771429 0.785714 0.8 0.814286 0.828571 0.842857 0.857143 0.871429 0.885714 0.9 0.914286 0.928571 0.942857 0.957143 0.971429 0.985714 1 1 1 1 1 1
  spline S27 degree 3 poles (29.5334, 35.9413) (29.5736, 35.9083) (29.6199, 35.8834) (29.7195, 35.8527) (29.7718, 35.8473) (29.8604, 35.8554) (29.8965, 35.8638) (29.9654, 35.8903) (29.9978, 35.9083) (30.0274, 35.9304) knots 0 0 0 0 0.015626 0.015626 0.031252 0.031252 0.042323 0.042323 0.053393 0.053393 0.053393 0.053393
  arc A14 (29.5334, 35.9413) -> (29.0156, 36.3606) centre (0, 0) ccw
  spline S28 degree 3 poles (28.9022, 36.8415) (28.8803, 36.7943) (28.8678, 36.7432) (28.8632, 36.6391) (28.871, 36.5872) (28.9011, 36.5034) (28.9183, 36.4706) (28.9612, 36.4105) (28.9868, 36.3836) (29.0156, 36.3606) knots 0 0 0 0 0.015626 0.015626 0.031252 0.031252 0.042323 0.042323 0.053393 0.053393 0.053393 0.053393
  spline S29 degree 5 poles (28.9022, 36.8415) (28.9028, 36.8428) (28.909, 36.8562) (28.9208, 36.8818) (28.9382, 36.9197) (28.9609, 36.97) (28.9883, 37.0315) (29.0153, 37.0932) (29.042, 37.1551) (29.0684, 37.2173) (29.0945, 37.2796) (29.1202, 37.3421) (29.1457, 37.4048) (29.1708, 37.4678) (29.1956, 37.5308) (29.2202, 37.5941) (29.2444, 37.6576) (29.2684, 37.7212) (29.2921, 37.785) (29.3155, 37.8489) (29.3386, 37.9131) (29.3615, 37.9774) (29.3841, 38.0418) (29.4064, 38.1064) (29.4284, 38.1712) (29.4502, 38.2361) (29.4717, 38.3012) (29.493, 38.3664) (29.514, 38.4317) (29.5348, 38.4972) (29.5553, 38.5629) (29.5755, 38.6287) (29.5955, 38.6946) (29.6153, 38.7607) (29.6348, 38.8269) (29.654, 38.8932) (29.673, 38.9597) (29.6918, 39.0263) (29.7103, 39.093) (29.7286, 39.1598) (29.7467, 39.2268) (29.7645, 39.2939) (29.7821, 39.3611) (29.7995, 39.4285) (29.8166, 39.496) (29.8335, 39.5635) (29.8502, 39.6313) (29.8666, 39.6991) (29.8829, 39.767) (29.8988, 39.8351) (29.9146, 39.9032) (29.9302, 39.9715) (29.9455, 40.0399) (29.9576, 40.0947) (29.9665, 40.1358) (29.9725, 40.1633) (29.9754, 40.177) knots 0.269981 0.269981 0.269981 0.269981 0.269981 0.269981 0.271429 0.285714 0.3 0.314286 0.328571 0.342857 0.357143 0.371429 0.385714 0.4 0.414286 0.428571 0.442857 0.457143 0.471429 0.485714 0.5 0.514286 0.528571 0.542857 0.557143 0.571429 0.585714 0.6 0.614286 0.628571 0.642857 0.657143 0.671429 0.685714 0.7 0.714286 0.728571 0.742857 0.757143 0.771429 0.785714 0.8 0.814286 0.828571 0.842857 0.857143 0.871429 0.885714 0.9 0.914286 0.928571 0.942857 0.957143 0.971429 0.985714 1 1 1 1 1 1
  arc A15 (29.9754, 40.177) -> (28.9477, 40.9237) centre (0, 0) ccw
  spline S30 degree 5 poles (26.1071, 38.8723) (26.1081, 38.8732) (26.119, 38.8833) (26.1397, 38.9025) (26.1704, 38.9307) (26.2112, 38.9678) (26.2612, 39.0128) (26.3115, 39.0576) (26.3622, 39.1022) (26.4131, 39.1465) (26.4643, 39.1905) (26.5158, 39.2343) (26.5676, 39.2779) (26.6197, 39.3213) (26.672, 39.3644) (26.7246, 39.4073) (26.7774, 39.4499) (26.8305, 39.4924) (26.8839, 39.5347) (26.9375, 39.5767) (26.9913, 39.6185) (27.0454, 39.6601) (27.0997, 39.7015) (27.1543, 39.7427) (27.2091, 39.7837) (27.2641, 39.8244) (27.3193, 39.865) (27.3747, 39.9054) (27.4304, 39.9456) (27.4863, 39.9855) (27.5424, 40.0253) (27.5987, 40.0649) (27.6552, 40.1043) (27.712, 40.1435) (27.7689, 40.1825) (27.826, 40.2213) (27.8834, 40.2599) (27.9409, 40.2984) (27.9986, 40.3366) (28.0566, 40.3747) (28.1147, 40.4126) (28.173, 40.4502) (28.2315, 40.4877) (28.2902, 40.5251) (28.3491, 40.5622) (28.4081, 40.5992) (28.4673, 40.6359) (28.5268, 40.6725) (28.5864, 40.709) (28.6461, 40.7452) (28.7061, 40.7813) (28.7662, 40.8171) (28.8265, 40.8529) (28.8749, 40.8813) (28.9112, 40.9025) (28.9355, 40.9166) (28.9477, 40.9237) knots 0.269981 0.269981 0.269981 0.269981 0.269981 0.269981 0.271429 0.285714 0.3 0.314286 0.328571 0.342857 0.357143 0.371429 0.385714 0.4 0.414286 0.428571 0.442857 0.457143 0.471429 0.485714 0.5 0.514286 0.528571 0.542857 0.557143 0.571429 0.585714 0.6 0.614286 0.628571 0.642857 0.657143 0.671429 0.685714 0.7 0.714286 0.728571 0.742857 0.757143 0.771429 0.785714 0.8 0.814286 0.828571 0.842857 0.857143 0.871429 0.885714 0.9 0.914286 0.928571 0.942857 0.957143 0.971429 0.985714 1 1 1 1 1 1
  spline S31 degree 3 poles (25.6147, 38.8315) (25.6582, 38.8028) (25.7068, 38.7829) (25.809, 38.7629) (25.8616, 38.7629) (25.9489, 38.7802) (25.9839, 38.7924) (26.0497, 38.8259) (26.0801, 38.8472) (26.1071, 38.8723) knots 0 0 0 0 0.015626 0.015626 0.031252 0.031252 0.042323 0.042323 0.053393 0.053393 0.053393 0.053393
  arc A16 (25.6147, 38.8315) -> (25.0559, 39.1944) centre (0, 0) ccw
  spline S32 degree 3 poles (24.8929, 39.6608) (24.876, 39.6115) (24.869, 39.5594) (24.8752, 39.4555) (24.8885, 39.4046) (24.9271, 39.3244) (24.9477, 39.2935) (24.9966, 39.2383) (25.0248, 39.2143) (25.0559, 39.1944) knots 0 0 0 0 0.015626 0.015626 0.031252 0.031252 0.042323 0.042323 0.053393 0.053393 0.053393 0.053393
  spline S33 degree 5 poles (24.8929, 39.6608) (24.8933, 39.6621) (24.8981, 39.6761) (24.9072, 39.7028) (24.9205, 39.7424) (24.9378, 39.7947) (24.9586, 39.8587) (24.9791, 39.923) (24.9991, 39.9873) (25.0189, 40.0519) (25.0383, 40.1166) (25.0574, 40.1815) (25.0761, 40.2465) (25.0946, 40.3117) (25.1127, 40.377) (25.1305, 40.4425) (25.148, 40.5081) (25.1651, 40.5739) (25.182, 40.6398) (25.1986, 40.7059) (25.2149, 40.7721) (25.2309, 40.8384) (25.2467, 40.9049) (25.2621, 40.9715) (25.2773, 41.0382) (25.2921, 41.105) (25.3067, 41.172) (25.3211, 41.2391) (25.3351, 41.3063) (25.3489, 41.3736) (25.3624, 41.441) (25.3757, 41.5085) (25.3887, 41.5762) (25.4014, 41.644) (25.4139, 41.7118) (25.4261, 41.7798) (25.4381, 41.8479) (25.4498, 41.9161) (25.4613, 41.9844) (25.4725, 42.0528) (25.4834, 42.1213) (25.4941, 42.1899) (25.5046, 42.2586) (25.5148, 42.3274) (25.5248, 42.3963) (25.5346, 42.4653) (25.5441, 42.5343) (25.5533, 42.6035) (25.5624, 42.6728) (25.5712, 42.7421) (25.5797, 42.8115) (25.588, 42.8811) (25.5961, 42.9507) (25.6024, 43.0064) (25.607, 43.0483) (25.6101, 43.0762) (25.6116, 43.0902) knots 0.269981 0.269981 0.269981 0.269981 0.269981 0.269981 0.271429 0.285714 0.3 0.314286 0.328571 0.342857 0.357143 0.371429 0.385714 0.4 0.414286 0.428571 0.442857 0.457143 0.471429 0.485714 0.5 0.514286 0.528571 0.542857 0.557143 0.571429 0.585714 0.6 0.614286 0.628571 0.642857 0.657143 0.671429 0.685714 0.7 0.714286 0.728571 0.742857 0.757143 0.771429 0.785714 0.8 0.814286 0.828571 0.842857 0.857143 0.871429 0.885714 0.9 0.914286 0.928571 0.942857 0.957143 0.971429 0.985714 1 1 1 1 1 1
  arc A17 (25.6116, 43.0902) -> (24.5114, 43.7254) centre (0, 0) ccw
  spline S34 degree 5 poles (21.9008, 41.3883) (21.9017, 41.3893) (21.9115, 41.4005) (21.9301, 41.4217) (21.9576, 41.453) (21.9943, 41.4942) (22.0394, 41.5442) (22.0848, 41.594) (22.1305, 41.6436) (22.1765, 41.6929) (22.2228, 41.7421) (22.2695, 41.7911) (22.3164, 41.8398) (22.3637, 41.8884) (22.4112, 41.9367) (22.459, 41.9849) (22.5071, 42.0328) (22.5555, 42.0806) (22.6041, 42.1282) (22.653, 42.1756) (22.7022, 42.2228) (22.7516, 42.2698) (22.8013, 42.3167) (22.8513, 42.3634) (22.9015, 42.4098) (22.9519, 42.4561) (23.0026, 42.5023) (23.0535, 42.5482) (23.1047, 42.594) (23.1561, 42.6396) (23.2077, 42.685) (23.2596, 42.7303) (23.3117, 42.7754) (23.364, 42.8203) (23.4166, 42.865) (23.4693, 42.9096) (23.5223, 42.954) (23.5755, 42.9982) (23.6289, 43.0423) (23.6826, 43.0862) (23.7364, 43.13) (23.7905, 43.1735) (23.8447, 43.2169) (23.8992, 43.2602) (23.9538, 43.3033) (24.0087, 43.3462) (24.0638, 43.389) (24.1191, 43.4316) (24.1745, 43.474) (24.2302, 43.5163) (24.286, 43.5585) (24.3421, 43.6004) (24.3983, 43.6422) (24.4434, 43.6756) (24.4774, 43.7005) (24.5001, 43.7171) (24.5114, 43.7254) knots 0.269981 0.269981 0.269981 0.269981 0.269981 0.269981 0.271429 0.285714 0.3 0.314286 0.328571 0.342857 0.357143 0.371429 0.385714 0.4 0.414286 0.428571 0.442857 0.457143 0.471429 0.485714 0.5 0.514286 0.528571 0.542857 0.557143 0.571429 0.585714 0.6 0.614286 0.628571 0.642857 0.657143 0.671429 0.685714 0.7 0.714286 0.728571 0.742857 0.757143 0.771429 0.785714 0.8 0.814286 0.828571 0.842857 0.857143 0.871429 0.885714 0.9 0.914286 0.928571 0.942857 0.957143 0.971429 0.985714 1 1 1 1 1 1
  spline S35 degree 3 poles (21.4154, 41.2963) (21.4616, 41.2723) (21.5121, 41.2576) (21.6158, 41.2483) (21.6681, 41.2539) (21.7531, 41.2802) (21.7867, 41.2959) (21.8486, 41.3362) (21.8766, 41.3605) (21.9008, 41.3883) knots 0 0 0 0 0.015626 0.015626 0.031252 0.031252 0.042323 0.042323 0.053393 0.053393 0.053393 0.053393
  arc A18 (21.4154, 41.2963) -> (20.8217, 41.5987) centre (0, 0) ccw
  spline S36 degree 3 poles (20.6108, 42.0456) (20.5992, 41.9948) (20.5977, 41.9422) (20.6147, 41.8395) (20.6332, 41.7903) (20.68, 41.7146) (20.7037, 41.686) (20.7582, 41.6362) (20.7887, 41.6152) (20.8217, 41.5987) knots 0 0 0 0 0.015626 0.015626 0.031252 0.031252 0.042323 0.042323 0.053393 0.053393 0.053393 0.053393
  spline S37 degree 5 poles (20.6108, 42.0456) (20.6112, 42.0469) (20.6144, 42.0613) (20.6207, 42.0889) (20.6298, 42.1295) (20.6415, 42.1834) (20.6555, 42.2493) (20.6691, 42.3153) (20.6824, 42.3814) (20.6953, 42.4476) (20.7078, 42.514) (20.72, 42.5805) (20.7319, 42.6472) (20.7434, 42.7139) (20.7545, 42.7808) (20.7654, 42.8478) (20.7759, 42.9149) (20.7862, 42.9821) (20.7961, 43.0495) (20.8057, 43.1169) (20.815, 43.1844) (20.8239, 43.2521) (20.8326, 43.3198) (20.841, 43.3876) (20.8491, 43.4556) (20.8569, 43.5236) (20.8645, 43.5917) (20.8717, 43.6599) (20.8787, 43.7282) (20.8853, 43.7966) (20.8917, 43.8651) (20.8979, 43.9336) (20.9037, 44.0023) (20.9093, 44.071) (20.9146, 44.1398) (20.9197, 44.2087) (20.9244, 44.2777) (20.929, 44.3467) (20.9332, 44.4158) (20.9372, 44.485) (20.941, 44.5543) (20.9444, 44.6237) (20.9477, 44.6931) (20.9507, 44.7626) (20.9534, 44.8321) (20.9559, 44.9017) (20.9581, 44.9714) (20.9601, 45.0412) (20.9618, 45.111) (20.9633, 45.1809) (20.9646, 45.2508) (20.9656, 45.3208) (20.9664, 45.3909) (20.9668, 45.447) (20.967, 45.4891) (20.9671, 45.5172) (20.9671, 45.5313) knots 0.269981 0.269981 0.269981 0.269981 0.269981 0.269981 0.271429 0.285714 0.3 0.314286 0.328571 0.342857 0.357143 0.371429 0.385714 0.4 0.414286 0.428571 0.442857 0.457143 0.471429 0.485714 0.5 0.514286 0.528571 0.542857 0.557143 0.571429 0.585714 0.6 0.614286 0.628571 0.642857 0.657143 0.671429 0.685714 0.7 0.714286 0.728571 0.742857 0.757143 0.771429 0.785714 0.8 0.814286 0.828571 0.842857 0.857143 0.871429 0.885714 0.9 0.914286 0.928571 0.942857 0.957143 0.971429 0.985714 1 1 1 1 1 1
  arc A19 (20.9671, 45.5313) -> (19.8066, 46.048) centre (0, 0) ccw
  spline S38 degree 5 poles (17.4546, 43.4508) (17.4554, 43.4519) (17.4639, 43.464) (17.4802, 43.4871) (17.5043, 43.5211) (17.5365, 43.5659) (17.5761, 43.6203) (17.616, 43.6746) (17.6563, 43.7287) (17.6969, 43.7826) (17.7378, 43.8363) (17.7791, 43.8899) (17.8207, 43.9433) (17.8626, 43.9965) (17.9048, 44.0496) (17.9474, 44.1025) (17.9902, 44.1552) (18.0333, 44.2078) (18.0767, 44.2602) (18.1204, 44.3125) (18.1644, 44.3645) (18.2086, 44.4165) (18.2531, 44.4683) (18.2979, 44.5199) (18.343, 44.5714) (18.3883, 44.6227) (18.4339, 44.6739) (18.4797, 44.7249) (18.5258, 44.7758) (18.5722, 44.8265) (18.6188, 44.8771) (18.6657, 44.9275) (18.7128, 44.9778) (18.7601, 45.0279) (18.8077, 45.0779) (18.8555, 45.1277) (18.9036, 45.1774) (18.9518, 45.227) (19.0004, 45.2764) (19.0491, 45.3257) (19.0981, 45.3748) (19.1473, 45.4238) (19.1967, 45.4727) (19.2463, 45.5214) (19.2962, 45.5699) (19.3463, 45.6184) (19.3966, 45.6666) (19.4471, 45.7148) (19.4978, 45.7628) (19.5487, 45.8107) (19.5999, 45.8584) (19.6512, 45.906) (19.7028, 45.9535) (19.7442, 45.9914) (19.7754, 46.0197) (19.7962, 46.0385) (19.8066, 46.048) knots 0.269981 0.269981 0.269981 0.269981 0.269981 0.269981 0.271429 0.285714 0.3 0.314286 0.328571 0.342857 0.357143 0.371429 0.385714 0.4 0.414286 0.428571 0.442857 0.457143 0.471429 0.485714 0.5 0.514286 0.528571 0.542857 0.557143 0.571429 0.585714 0.6 0.614286 0.628571 0.642857 0.657143 0.671429 0.685714 0.7 0.714286 0.728571 0.742857 0.757143 0.771429 0.785714 0.8 0.814286 0.828571 0.842857 0.857143 0.871429 0.885714 0.9 0.914286 0.928571 0.942857 0.957143 0.971429 0.985714 1 1 1 1 1 1
  spline S39 degree 3 poles (16.9814, 43.3086) (17.0299, 43.2895) (17.0816, 43.2802) (17.1858, 43.2818) (17.2372, 43.2928) (17.319, 43.3279) (17.3507, 43.347) (17.4081, 43.3935) (17.4334, 43.4206) (17.4546, 43.4508) knots 0 0 0 0 0.015626 0.015626 0.031252 0.031252 0.042323 0.042323 0.053393 0.053393 0.053393 0.053393
  arc A20 (16.9814, 43.3086) -> (16.3594, 43.5473) centre (0, 0) ccw
  spline S40 degree 3 poles (16.103, 43.9697) (16.0967, 43.918) (16.1007, 43.8655) (16.1284, 43.7651) (16.1519, 43.7181) (16.2064, 43.6477) (16.2329, 43.6218) (16.2923, 43.578) (16.3249, 43.5603) (16.3594, 43.5473) knots 0 0 0 0 0.015626 0.015626 0.031252 0.031252 0.042323 0.042323 0.053393 0.053393 0.053393 0.053393
  spline S41 degree 5 poles (16.103, 43.9697) (16.1031, 43.971) (16.1049, 43.9857) (16.1082, 44.0137) (16.113, 44.0551) (16.1191, 44.11) (16.1261, 44.1769) (16.1328, 44.244) (16.139, 44.3111) (16.1449, 44.3784) (16.1504, 44.4457) (16.1556, 44.5131) (16.1604, 44.5806) (16.1649, 44.6482) (16.169, 44.7159) (16.1728, 44.7837) (16.1763, 44.8515) (16.1794, 44.9194) (16.1823, 44.9874) (16.1847, 45.0555) (16.1869, 45.1236) (16.1888, 45.1918) (16.1904, 45.2601) (16.1916, 45.3284) (16.1926, 45.3968) (16.1932, 45.4653) (16.1936, 45.5338) (16.1937, 45.6024) (16.1934, 45.6711) (16.1929, 45.7398) (16.1921, 45.8086) (16.1911, 45.8774) (16.1897, 45.9463) (16.1881, 46.0152) (16.1862, 46.0842) (16.184, 46.1532) (16.1815, 46.2223) (16.1788, 46.2915) (16.1758, 46.3606) (16.1726, 46.4299) (16.169, 46.4992) (16.1653, 46.5685) (16.1612, 46.6379) (16.1569, 46.7073) (16.1524, 46.7767) (16.1476, 46.8462) (16.1425, 46.9158) (16.1372, 46.9854) (16.1316, 47.055) (16.1258, 47.1246) (16.1197, 47.1943) (16.1134, 47.2641) (16.1069, 47.3338) (16.1014, 47.3897) (16.0972, 47.4316) (16.0944, 47.4595) (16.093, 47.4735) knots 0.269981 0.269981 0.269981 0.269981 0.269981 0.269981 0.271429 0.285714 0.3 0.314286 0.328571 0.342857 0.357143 0.371429 0.385714 0.4 0.414286 0.428571 0.442857 0.457143 0.471429 0.485714 0.5 0.514286 0.528571 0.542857 0.557143 0.571429 0.585714 0.6 0.614286 0.628571 0.642857 0.657143 0.671429 0.685714 0.7 0.714286 0.728571 0.742857 0.757143 0.771429 0.785714 0.8 0.814286 0.828571 0.842857 0.857143 0.871429 0.885714 0.9 0.914286 0.928571 0.942857 0.957143 0.971429 0.985714 1 1 1 1 1 1
  arc A21 (16.093, 47.4735) -> (14.8847, 47.8661) centre (0, 0) ccw
  spline S42 degree 5 poles (12.8171, 45.0373) (12.8178, 45.0385) (12.825, 45.0514) (12.8388, 45.076) (12.8593, 45.1124) (12.8866, 45.1603) (12.9202, 45.2186) (12.9543, 45.2767) (12.9887, 45.3347) (13.0234, 45.3926) (13.0585, 45.4503) (13.094, 45.5079) (13.1298, 45.5654) (13.1659, 45.6227) (13.2023, 45.6798) (13.2391, 45.7369) (13.2762, 45.7938) (13.3135, 45.8506) (13.3512, 45.9073) (13.3892, 45.9638) (13.4275, 46.0202) (13.4661, 46.0765) (13.5049, 46.1326) (13.5441, 46.1887) (13.5835, 46.2446) (13.6232, 46.3003) (13.6632, 46.356) (13.7035, 46.4115) (13.744, 46.4669) (13.7848, 46.5222) (13.8259, 46.5774) (13.8672, 46.6325) (13.9088, 46.6874) (13.9506, 46.7422) (13.9927, 46.7969) (14.0351, 46.8515) (14.0777, 46.9059) (14.1205, 46.9602) (14.1636, 47.0145) (14.2069, 47.0686) (14.2505, 47.1225) (14.2943, 47.1764) (14.3383, 47.2301) (14.3826, 47.2838) (14.4271, 47.3373) (14.4719, 47.3907) (14.5169, 47.444) (14.5621, 47.4971) (14.6075, 47.5502) (14.6531, 47.6031) (14.699, 47.656) (14.7451, 47.7087) (14.7914, 47.7613) (14.8286, 47.8032) (14.8567, 47.8347) (14.8754, 47.8556) (14.8847, 47.8661) knots 0.269981 0.269981 0.269981 0.269981 0.269981 0.269981 0.271429 0.285714 0.3 0.314286 0.328571 0.342857 0.357143 0.371429 0.385714 0.4 0.414286 0.428571 0.442857 0.457143 0.471429 0.485714 0.5 0.514286 0.528571 0.542857 0.557143 0.571429 0.585714 0.6 0.614286 0.628571 0.642857 0.657143 0.671429 0.685714 0.7 0.714286 0.728571 0.742857 0.757143 0.771429 0.785714 0.8 0.814286 0.828571 0.842857 0.857143 0.871429 0.885714 0.9 0.914286 0.928571 0.942857 0.957143 0.971429 0.985714 1 1 1 1 1 1